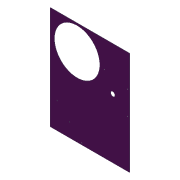
# Autodesk Inventor part: Shooter Plate
Saved by Autodesk Inventor 2012 (Build 160160000, 160)
## iProperties
Created: 2013-01-15
Part Number: Shooter Plate
Material: Default
Document SubType Name: Modeling
Designer: William
Density: 1 g/cm^3
Mass: 424.878 g
Surface Area: 5407.79 cm^2
Volume: 424.878 cm^3
Author: William
Autodesk Inventor part; units mm, degrees
ref_plane "YZ Plane" through (0, 0, 0) normal (1, 0, 0) x (0, 1, 0)
ref_plane "XZ Plane" through (0, 0, 0) normal (0, 1, 0) x (-1, 0, 0)
ref_plane "XY Plane" through (0, 0, 0) normal (0, 0, 1) x (1, 0, 0)
sketch "Sketch1" plane through (0, 0, 0) normal (0, 0, 1) x (1, 0, 0)
  line L0 (-254, -330.2) -> (254, -330.2)
  line L1 (254, -330.2) -> (254, 330.2)
  line L2 (254, 330.2) -> (-254, 330.2)
  line L3 (-254, 330.2) -> (-254, -330.2)
  point P0 (0, 0)
  dimension "d0" = 508
  dimension "d1" = 660.4
  dimension "d2" = 330.2
  dimension "d3" = 254
  constraints: 8 end point, 2 parallel, 1 horizontal, 1 perpendicular
  measures "d0" distance of L1.end L2.end
  measures "d1" distance of L2.end L0.start
  measures "d2" distance from line of L2 point (0, 0)
  measures "d3" distance from line of L3 point (0, 0)
extrude "Extrusion1" add sketch "Sketch1" along normal blind 1.5875
sketch "Sketch2" plane through (0, 0, 1.5875) normal (0, 0, 1) x (1, 0, 0)
  line L0 (-254, -330.2) -> (-254, 330.2) projected
  line L1 (254, -330.2) -> (-254, -330.2) projected
  line L2 (-254, 330.2) -> (254, 330.2) projected
  circle A0 centre (-82.55, 171.45) radius 146.05
  circle A1 centre (146.05, 50.8) radius 95.25
  arc A2 (-228.6, 50.8) -> (146.05, -323.85) centre (146.05, 50.8) ccw
  line L3 (-228.6, 50.8) -> (-228.6, 203.2)
  line L4 (146.05, -323.85) -> (222.25, -323.85)
  circle A3 centre (146.05, 50.8) radius 14.2875
  circle A4 centre (76.4372, 288.4526) radius 3.175
  circle A5 centre (171.4841, 288.4526) radius 3.175
  line L5 (254, 330.2) -> (254, -330.2) projected
  point P0 (0, 0)
  point P1 (-82.55, 317.5)
  point P2 (-10.4279, 298.45)
  dimension "d6" = 292.1
  dimension "d7" = 158.75
  dimension "d8" = 171.45
  dimension "d11" = 190.5
  dimension "d16" = 152.4
  dimension "d19" = 76.2
  dimension "d23" = 28.575
  dimension "d27" = 279.4
  dimension "d28" = 25.4
  dimension "d29" = 6.35
  dimension "d31" = 381
  dimension "d33" = 6.35
  dimension "d34" = 6.35
  dimension "d215" = 107.95
  constraints: 6 centre point, 4 end point, 4 point on circle, 2 coincident, 2 tangent, 1 perpendicular
  measures "d6" diameter of A0
  measures "d7" distance from line of L2 A0.centre
  measures "d8" distance from line of L0 A0.centre
  measures "d11" diameter of A1
  measures "d16" distance of L3.start L3.end
  measures "d19" distance of L4.start L4.end
  measures "d23" diameter of A3
  measures "d27" radial gap between concentric circles of A2 A1
  measures "d28" distance between parallel lines of L0 L3
  measures "d29" distance between parallel lines of L1 L4
  measures "d31" distance from line of L1 A1.centre
  measures "d33" diameter of A4
  measures "d34" diameter of A5
  measures "d215" distance from line of L5 A3.centre
extrude "Extrusion2" cut sketch "Sketch2" against normal blind 93.6625 contours A0 | A3
sketch "Sketch10" plane through (0, 0, 1.5875) normal (0, 0, 1) x (1, 0, 0)
  circle A0 centre (146.05, 50.8) radius 14.2875 projected
  line L0 (254, 330.2) -> (254, -330.2) projected
  circle A1 centre (241.3, 127) radius 3.175
  circle A2 centre (241.3, -25.4) radius 3.175
  circle A3 centre (92.6171, 160.4537) radius 3.175
  line L1 (241.3, -25.4) -> (241.3, 127) construction
  line L2 (241.3, 127) -> (92.6171, 160.4537) construction
  line L3 (146.05, 50.8) -> (241.3, -25.4) construction
  line L4 (146.05, 50.8) -> (241.3, 127) construction
  line L5 (146.05, 50.8) -> (92.6171, 160.4537) construction
  point P0 (0, 0)
  dimension "d208" = 6.35
  dimension "d210" = 12.7
  dimension "d214" = 152.4
  constraints: 10 end point, 3 centre point, 3 equal length, 2 equal radius, 1 vertical
  measures "d208" diameter of A1
  measures "d210" distance from line of L0 L1.start
  measures "d214" distance of L1.start L1.end
extrude "Extrusion10" cut sketch "Sketch10" against normal up to next contours A1 | A2 | A3
sketch "Sketch11" plane through (0, 0, 1.5875) normal (0, 0, 1) x (1, 0, 0)
  line L0 (-254, -330.2) -> (-254, 330.2) projected
  line L1 (254, -330.2) -> (-254, -330.2) projected
  line L2 (-254, -330.2) -> (-254, -171.45) construction
  line L3 (-254, -171.45) -> (-95.25, -330.2) construction
  line L4 (-254, -330.2) -> (-95.25, -330.2) construction
  circle A0 centre (-209.0987, -162.4697) radius 3.175
  circle A1 centre (-130.1559, -241.4125) radius 3.175
  circle A2 centre (-51.2132, -320.3553) radius 3.175
  line L5 (-209.0987, -162.4697) -> (-130.1559, -241.4125) construction
  line L6 (-130.1559, -241.4125) -> (-51.2132, -320.3553) construction
  line L7 (-254, -171.45) -> (-217.3278, -134.7778) construction
  point P0 (0, 0)
  dimension "d216" = 158.75
  dimension "d217" = 158.75
  dimension "d218" = 6.35
  dimension "d219" = 38.1
  dimension "d220" = 25.4
  constraints: 12 end point, 3 centre point, 2 collinear, 2 equal radius, 2 point on line, 1 horizontal, 1 parallel, 1 perpendicular
  measures "d216" distance of L0.start L2.end
  measures "d217" distance of L0.start L3.end
  measures "d218" diameter of A1
  measures "d219" distance between parallel lines of L5 L3
  measures "d220" distance from line of L5.start L7
extrude "Extrusion11" cut sketch "Sketch11" against normal up to next
equation "\"d2\" = 0.5 * d1"
equation "\"d3\" = 0.5 * d0"
body "Solid1"
